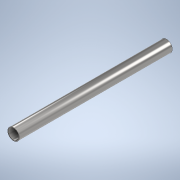
# Autodesk Inventor part: strut
Saved by Autodesk Inventor 2020.2 (Build 242310000, 310)
## iProperties
Created: 2020-03-22
Part Number: strut
Material: Steel, Galvanized
Document SubType Name: Modeling
Designer: agmle
Density: 7.85 g/cm^3
Appearance: Galvanized
Author: agmle
Autodesk Inventor part; units mm, degrees
ref_plane "YZ Plane" through (0, 0, 0) normal (1, 0, 0) x (0, 1, 0)
ref_plane "XZ Plane" through (0, 0, 0) normal (0, 1, 0) x (-1, 0, 0)
ref_plane "XY Plane" through (0, 0, 0) normal (0, 0, 1) x (1, 0, 0)
sketch "Sketch1" plane through (0, 0, 0) normal (0, 0, 1) x (1, 0, 0)
  circle A0 centre (0, 0) radius 13.3223
  circle A1 centre (0, 0) radius 14.7701
  dimension "d0" = 29.5402
  dimension "d1" = 1.4478
  constraints: 2 centre point, 2 coincident
  measures "d0" diameter of A1
  measures "d1" radial gap between concentric circles of A1 A0
extrude "Extrusion1" add sketch "Sketch1" along normal blind 390.525
equation "\"d2\" = hull_spacing"
equation "\"hull_od\" = 219.075"
equation "\"hull_id\" = 201.7268"
equation "\"hull_wall\" = 8.6741"
equation "\"hull_length\" = 609.6"
equation "\"hull_spacing\" = 390.525"
equation "\"impeller_od\" = 76.2"
equation "\"impeller_clearance\" = 0.5"
equation "\"impeller_shaft_id\" = 3.175"
equation "\"impeller_shaft_od\" = 5.715"
equation "\"impeller_shaft_support\" = 3.175"
equation "\"impeller_intake_od\" = 19.05"
equation "\"impeller_vane_thick\" = 2"
equation "\"impeller_vane_inner_rad\" = 3.175"
equation "\"impeller_vane_outer_rad\" = 0.37206"
equation "\"magnet_od\" = 5.95"
equation "\"magnet_clearance\" = 0.25"
equation "\"magnet_rad\" = 0.25"
equation "\"magnet_circle_offset\" = 3.175"
equation "\"motor_shaft_od\" = 12.7"
equation "\"motor_shaft_length\" = 31.75"
equation "\"motor_shaft_key\" = 3.048"
body "Solid1"
